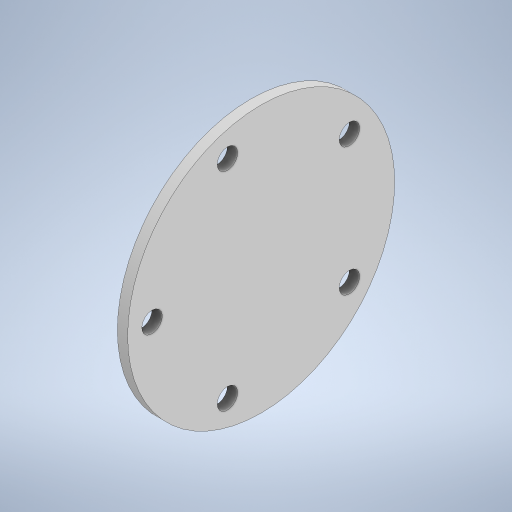
# Autodesk Inventor part: antenna_plate
Saved by Autodesk Inventor 2024 (Build 280153000, 153)
## iProperties
Created: 2025-12-27
Part Number: antenna_plate
Material: Generic
Document SubType Name: Modeling
Designer: schar
Density: 1 g/cm^3
Appearance: Default
Author: schar
Autodesk Inventor part; units mm, degrees
ref_plane "YZ Plane" through (0, 0, 0) normal (1, 0, 0) x (0, 1, 0)
ref_plane "XZ Plane" through (0, 0, 0) normal (0, 1, 0) x (-1, 0, 0)
ref_plane "XY Plane" through (0, 0, 0) normal (0, 0, 1) x (1, 0, 0)
sketch "Sketch1" plane through (0, 0, 0) normal (1, 0, 0) x (0, 1, 0)
  circle A0 centre (0, 0) radius 21.25
  circle A1 centre (0, 0) radius 26
  circle A2 centre (0, 21.25) radius 2
  circle A3 centre (-20.21, 6.5666) radius 2
  circle A4 centre (-12.4904, -17.1916) radius 2
  circle A5 centre (12.4904, -17.1916) radius 2
  circle A6 centre (20.21, 6.5666) radius 2
  dimension "d0" = 42.5
  dimension "d1" = 52
  dimension "d2" = 4
  dimension "d5" = 360
  constraints: 6 centre point, 2 coincident, 1 vertical alignment, 13 other
  measures "d1" diameter of A1
  measures "d2" diameter of A2
extrude "Extrusion1" add sketch "Sketch1" along normal blind 2 contours A0 A5 A4 A3 A2 A6 | A1
body "Solid1"
